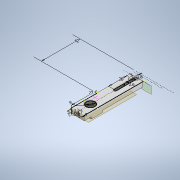
# Autodesk Inventor part: Sensor_Montage
Saved by Autodesk Inventor 2022 (Build 260153000, 153)
## iProperties
Created: 2024-04-03
Part Number: Sensor_Montage
Material: Generic
Document SubType Name: Modeling
Designer: Gotham City
Density: 1 g/cm^3
Appearance: Default
Author: Gotham City
Autodesk Inventor part; units mm, degrees
ref_plane "YZ Plane" through (0, 0, 0) normal (1, 0, 0) x (0, 1, 0)
ref_plane "XZ Plane" through (0, 0, 0) normal (0, 1, 0) x (-1, 0, 0)
ref_plane "XY Plane" through (0, 0, 0) normal (0, 0, 1) x (1, 0, 0)
sketch "Sketch1" plane through (0, 0, 0) normal (1, 0, 0) x (0, 1, 0)
  line L0 (0, 13.75) -> (-5.2, 13.75)
  line L1 (-5.2, 13.75) -> (-5.2, 6.2)
  line L2 (-5.2, 6.2) -> (-7.4, 6.2)
  line L3 (-7.4, 6.2) -> (-7.4, 2.5)
  line L4 (-7.4, 2.5) -> (-13.4, 2.5) construction
  line L5 (-13.4, 2.5) -> (-13.4, -1.6142) construction
  line L6 (-16.08, 0) -> (2.68, 0) construction
  line L7 (0, -13.75) -> (-5.2, -13.75)
  line L8 (-5.2, -13.75) -> (-5.2, -6.2)
  line L9 (-5.2, -6.2) -> (-7.4, -6.2)
  line L10 (-7.4, -6.2) -> (-7.4, -2.5)
  line L11 (-7.4, -2.5) -> (-13.4, -2.5) construction
  line L12 (-13.4, -2.5) -> (-13.4, -1.6142) construction
  line L13 (0, 13.75) -> (0, -13.75)
  line L14 (-7.4, 2.5) -> (-7.4, -2.5)
  point P0 (0, 0)
  dimension "d1" = 5
  dimension "d2" = 3.7
  dimension "d3" = 6
  dimension "d4" = 2.2
  dimension "d5" = 5.2
  dimension "d52" = 27.5
  dimension "d53" = 7.55
  constraints: 28 end point, 6 perpendicular, 6 vertical alignment, 1 horizontal, 1 midpoint, 1 parallel, 1 other
  measures "d1" distance of L11.end L4.end
  measures "d2" distance of L2.end L3.end
  measures "d3" distance of L3.end L4.end
  measures "d4" distance of L1.end L2.end
  measures "d5" distance of L0.start L0.end
  measures "d52" distance between parallel lines of L7 L0
  measures "d53" distance of L0.end L1.end
extrude "Extrusion1" add sketch "Sketch1" along normal blind 14
sketch "Sketch2" plane through (0, -5.2, -13.75) normal (0, 0, -1) x (-1, 0, 0)
  line L0 (0, 0) -> (0, 5.2) projected
  line L1 (0, 5.2) -> (-14, 5.2) projected
  line L2 (-14, 0) -> (-14, 5.2) projected
  line L3 (0, 0) -> (-14, 0) projected
  point P0 (0, 5.2)
sketch "Sketch3" plane through (0, 0, 13.75) normal (0, 1, 0) x (1, 0, 0)
  line L0 (0, 0) -> (14, 0) construction
  line L1 (7, 40.444) -> (7, 60.444) construction
  line L2 (5.7, 40.444) -> (5.7, 60.444)
  line L3 (8.3, 60.444) -> (8.3, 40.444)
  arc A0 (5.7, 40.444) -> (8.3, 40.444) centre (7, 40.444) ccw
  arc A1 (8.3, 60.444) -> (5.7, 60.444) centre (7, 60.444) ccw
  line L4 (0, 69.5) -> (41.7053, 69.5) construction
  circle A2 centre (7, 61.2) radius 2.5 construction
  line L5 (0, 63.7) -> (21.4479, 63.7) construction
  line L6 (-0.0005, 67.5) -> (30.8862, 67.5) construction
  line L7 (0, 27.5) -> (0, 0) construction
  line L8 (7, 0) -> (7, 40.444) construction
  point P0 (7, 50.444)
  dimension "d55" = 2.6
  dimension "d57" = 42
  dimension "d58" = 0.756
  dimension "d59" = 5
  dimension "d60" = 3.8
  dimension "d61" = 2
  dimension "d62" = 20
  constraints: 16 end point, 5 tangent, 4 point on circle, 3 centre point, 3 horizontal, 2 midpoint, 2 vertical, 1 parallel, 1 point on line
  measures "d55" distance between parallel lines of L3 L2
  measures "d57" distance from line of L4 L7.start
  measures "d58" distance of A2.centre L1.end
  measures "d59" diameter of A2
  measures "d60" distance between parallel lines of L6 L5
  measures "d61" distance between parallel lines of L4 L6
  measures "d62" distance of L1.start L1.end
ref_plane "Work Plane2" through (0, 0, -49.95) normal (0, 0, -1) x (-1, 0, 0)
extrude "Extrusion8" add sketch "Sketch2" along normal up to surface (36.2 mm away)
extrude "Extrusion7" cut sketch "Sketch3" against normal through all
sketch "Sketch5" plane through (0, 0, 13.75) normal (0, 1, 0) x (1, 0, 0)
  point P0 (0, 13.75)
ref_plane "Work Plane1" through (0, -2, 13.75) normal (0, 1, 0) x (1, 0, 0)
sketch "Sketch7" plane through (0, 0, 13.75) normal (0, 1, 0) x (1, 0, 0)
  line L0 (18.6924, 13.75) -> (-14.1545, 13.75) construction
  circle A0 centre (7, 13.75) radius 4.5
  line L1 (14, 0) -> (14, 63.7)
  line L2 (0, 0) -> (14, 0) construction
  line L3 (14, 63.7) -> (-7.462, 63.7) construction
  line L4 (7, 0) -> (7, 13.75) construction
  point P0 (0, 13.75)
  point P1 (3.3, 22.5)
  dimension "d24" = 9
  constraints: 6 end point, 1 centre point, 1 coincident, 1 midpoint, 1 vertical, 2 other
  measures "d24" diameter of A0
hole "Hole1" at (7, 0, 0) direction (0, -1, 0) diameter 5.5 end through all counterbore diameter 10 counterbore depth 5 clearance for "Socket Head Cap Screw ISO 4762" size "M5" standard "ISO"
body "Solid1"
